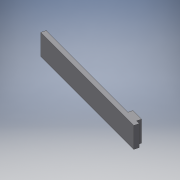
# Autodesk Inventor part: Spring
Saved by Autodesk Inventor 2016 SP2 (Build 200236200, 236)
## iProperties
Created: 2018-09-27
Part Number: Spring
Material: Generisch
Document SubType Name: Modeling
Designer: Nils
Density: 1 g/cm^3
Appearance: Vorgabe
Author: Nils
Autodesk Inventor part; units mm, degrees
ref_plane "YZ Plane" through (0, 0, 0) normal (1, 0, 0) x (0, 1, 0)
ref_plane "XZ Plane" through (0, 0, 0) normal (0, 1, 0) x (-1, 0, 0)
ref_plane "XY Plane" through (0, 0, 0) normal (0, 0, 1) x (1, 0, 0)
sketch "Skizze1" plane through (0, 0, 0) normal (0, 0, 1) x (1, 0, 0)
  line L0 (52.7974, -26.0018) -> (57.627, -27.2959) projected
  line L1 (52.3833, -27.5473) -> (52.7974, -26.0018) projected
  line L2 (57.627, -27.2959) -> (57.2129, -28.8414) projected
  line L3 (58.6618, -29.2296) -> (58.1442, -31.1615) projected
  line L4 (57.2129, -28.8414) -> (58.6618, -29.2296) projected
  line L5 (58.1442, -31.1615) -> (8.882, -17.9617)
  line L6 (8.882, -17.9617) -> (9.3996, -16.0299)
  line L7 (9.3996, -16.0299) -> (52.3833, -27.5473)
  line L8 (9.0657, -17.8557) -> (58.0381, -30.9778)
  line L9 (58.0381, -30.9778) -> (58.4781, -29.3357)
  line L10 (58.4781, -29.3357) -> (57.0292, -28.9475)
  line L11 (57.0292, -28.9475) -> (57.4433, -27.402)
  line L12 (57.4433, -27.402) -> (52.9035, -26.1856)
  line L13 (52.9035, -26.1856) -> (52.4894, -27.731)
  line L14 (52.4894, -27.731) -> (9.5057, -16.2136)
  line L15 (9.5057, -16.2136) -> (9.0657, -17.8557)
  point P0 (0, 0)
  dimension "d0" = 51
  dimension "d2" = 2
  dimension "d5" = 0.15
  constraints: 22 end point, 2 parallel, 2 perpendicular, 7 other
  measures "d0" distance of L3.end L5.end
  measures "d2" distance of L5.end L6.end
  measures "d5" distance between parallel lines of L8 L5
extrude "Extrusion1" add sketch "Skizze1" against normal blind 8 contours L15 L14 L13 L12 L11 L10 L9 L8
